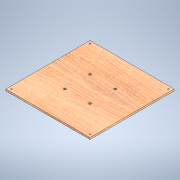
# Autodesk Inventor part: Base_Mdf
Saved by Autodesk Inventor 2022 (Build 260153000, 153)
## iProperties
Created: 2022-01-24
Part Number: Base_Mdf
Material: Wood (Birch)
Document SubType Name: Modeling
Designer: hurta
Density: 0.55 g/cm^3
Appearance: Birch - Natural Polished
Author: hurta
Autodesk Inventor part; units mm, degrees
ref_plane "YZ Plane" through (0, 0, 0) normal (1, 0, 0) x (0, 1, 0)
ref_plane "XZ Plane" through (0, 0, 0) normal (0, 1, 0) x (-1, 0, 0)
ref_plane "XY Plane" through (0, 0, 0) normal (0, 0, 1) x (1, 0, 0)
sketch "Sketch1" plane through (0, 0, 0) normal (0, 1, 0) x (-1, 0, 0)
  line L0 (150, -150) -> (-150, -150)
  line L1 (-150, -150) -> (-150, 150)
  line L2 (-150, 150) -> (150, 150)
  line L3 (150, 150) -> (150, -150)
  line L4 (150, -150) -> (-150, 150) construction
  line L5 (-150, -150) -> (150, 150) construction
  point P0 (0, 0)
  point P1 (45, 45)
  point P2 (-45, 45)
  point P3 (-45, -45)
  point P4 (45, -45)
  dimension "d0" = 300
  dimension "d1" = 300
  dimension "d2" = 45
  dimension "d4" = 45
  dimension "d5" = 45
  dimension "d6" = 45
  constraints: 12 end point, 2 horizontal alignment, 2 midpoint, 2 parallel, 2 vertical alignment, 1 horizontal, 1 perpendicular
  measures "d0" distance of L1.end L2.end
  measures "d1" distance of L0.end L1.end
  measures "d2" horizontal distance of point (45, 45) point (0, 0)
  measures "d4" horizontal distance of point (0, 0) point (45, 45)
  measures "d5" horizontal distance of point (0, 0) point (-45, -45)
  measures "d6" horizontal distance of point (0, 0) point (-45, -45)
extrude "Extrusion1" add sketch "Sketch1" along normal blind 6.2
hole "Hole1" at (-45, 0, 45) at (45, 0, 45) at (45, 0, -45) at (-45, 0, -45) direction (0, 1, 0) diameter 8.35 end through all
sketch "Sketch2" plane through (0, 6.2, 0) normal (0, 1, 0) x (1, 0, 0)
  line L0 (-150, -150) -> (150, -150) projected
  line L1 (-150, 150) -> (-150, -150) projected
  line L2 (150, 150) -> (-150, 150) projected
  line L3 (150, -150) -> (150, 150) projected
  point P0 (0, 0)
  point P1 (-140, -140)
  point P2 (140, -140)
  point P3 (140, 140)
  point P4 (-140, 140)
  dimension "d16" = 10
  dimension "d17" = 10
  dimension "d18" = 10
  dimension "d19" = 10
  constraints: 2 horizontal alignment, 2 vertical alignment
  measures "d16" distance from line of L0 point (-140, -140)
  measures "d17" distance from line of L1 point (-140, -140)
  measures "d18" distance from line of L2 point (140, 140)
  measures "d19" distance from line of L3 point (140, 140)
hole "Hole2" at (140, 6.2, 140) at (140, 6.2, -140) at (-140, 6.2, -140) at (-140, 6.2, 140) direction (0, -1, 0) diameter 4.5 end through all
body "Solid1"
